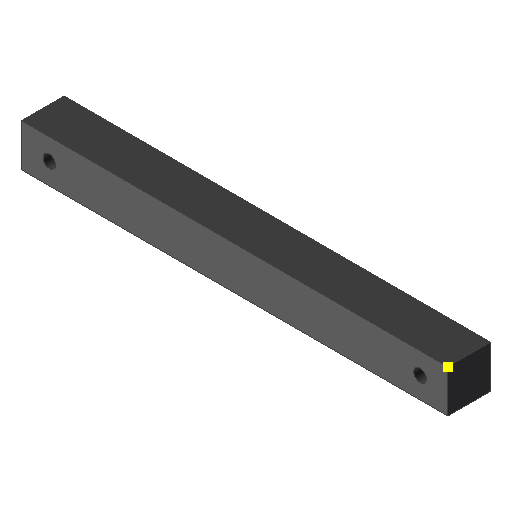
# Autodesk Inventor part: fengmingroboticarm1
Saved by Autodesk Inventor 2025 (Build 290162000, 162)
## iProperties
Created: 2025-02-16
Part Number: fengmingroboticarm1
Material: Generic
Document SubType Name: Modeling
Designer: wj
Density: 1 g/cm^3
Appearance: Default
Author: wj
Autodesk Inventor part; units mm, degrees
ref_plane "YZ Plane" through (0, 0, 0) normal (1, 0, 0) x (0, 1, 0)
ref_plane "XZ Plane" through (0, 0, 0) normal (0, 1, 0) x (-1, 0, 0)
ref_plane "XY Plane" through (0, 0, 0) normal (0, 0, 1) x (1, 0, 0)
sketch "Sketch1" plane through (0, 0, 0) normal (1, 0, 0) x (0, 1, 0)
  line L0 (0, 0) -> (-10, 0)
  line L1 (-10, 0) -> (-10, -10)
  line L2 (-10, -10) -> (0, -10)
  line L3 (0, -10) -> (0, 0)
  dimension "d0" = 10
  dimension "d1" = 10
  constraints: 8 end point, 2 parallel, 1 horizontal, 1 perpendicular
  measures "d0" distance of L2.end L0.start
  measures "d1" distance of L1.end L2.end
extrude "Extrusion1" add sketch "Sketch1" along normal blind 100
sketch "Sketch2" plane through (100, 0, 0) normal (1, 0, 0) x (0, 0, -1)
  point P0 (0, 0)
sketch "Sketch3" plane through (0, -10, 0) normal (0, 0, 1) x (1, 0, 0)
  circle A0 centre (6.5, 5) radius 1.5
  circle A1 centre (93.5, 5) radius 1.5
  line L0 (0, 0) -> (0, 10) projected
  line L1 (100, 10) -> (100, 0) projected
  line L2 (0, 0) -> (100, 0) projected
  dimension "d4" = 3
  dimension "d5" = 3
  dimension "d6" = 5
  dimension "d7" = 5
  dimension "d8" = 3.5
  dimension "d9" = 5
  constraints: 2 centre point
  measures "d4" diameter of A0
  measures "d5" diameter of A1
  measures "d6" distance edge to line of A0 L0
  measures "d7" distance edge to line of A1 L1
  measures "d8" distance edge to line of A0 L2
  measures "d9" distance from line of L2 A1.centre
extrude "Extrusion2" cut sketch "Sketch3" against normal blind 100
body "Solid1"
